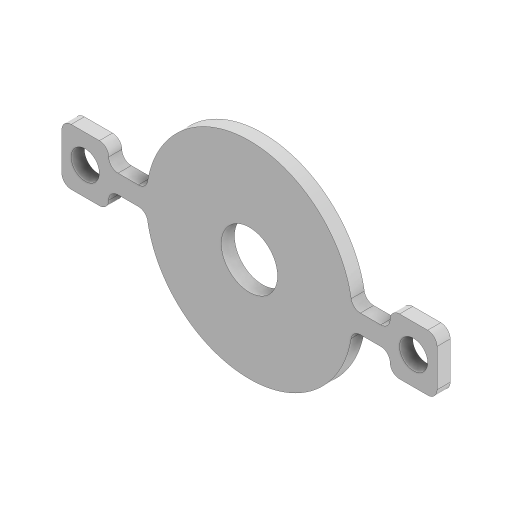
# Autodesk Inventor part: TAPA QUE DESPLAZA CON TORNILLOS
Saved by Autodesk Inventor 2024 (Build 280153000, 153)
## iProperties
Created: 2024-05-26
Part Number: TAPA QUE DESPLAZA CON TORNILLOS
Material: Generic
Document SubType Name: Modeling
Designer: Jhuliams
Density: 1 g/cm^3
Appearance: Default
Author: Jhuliams
Autodesk Inventor part; units mm, degrees
ref_plane "YZ Plane" through (0, 0, 0) normal (1, 0, 0) x (0, 1, 0)
ref_plane "XZ Plane" through (0, 0, 0) normal (0, 1, 0) x (-1, 0, 0)
ref_plane "XY Plane" through (0, 0, 0) normal (0, 0, 1) x (1, 0, 0)
sketch "Sketch1" plane through (0, 0, 0) normal (0, 0, 1) x (1, 0, 0)
  circle A0 centre (0, 0) radius 55
  line L0 (100, 15) -> (100, -15)
  line L1 (10, -15) -> (10, 15)
  line L2 (10, 15) -> (100, -15) construction
  line L3 (100, 15) -> (10, -15) construction
  line L4 (0, 0) -> (0, 20) construction
  line L5 (-100, 15) -> (-100, -15)
  line L6 (-10, -15) -> (-10, 15)
  line L7 (-10, 15) -> (-100, -15) construction
  line L8 (-100, 15) -> (-10, -15) construction
  line L9 (-75, 5) -> (-35, 5)
  line L10 (-35, 5) -> (-35, -5)
  line L11 (-35, -5) -> (-75, -5)
  line L12 (-75, -5) -> (-75, 5)
  line L13 (-75, 5) -> (-35, -5) construction
  line L14 (-35, 5) -> (-75, -5) construction
  line L15 (75, 5) -> (35, 5)
  line L16 (35, 5) -> (35, -5)
  line L17 (35, -5) -> (75, -5)
  line L18 (75, -5) -> (75, 5)
  line L19 (75, 5) -> (35, -5) construction
  line L20 (35, 5) -> (75, -5) construction
  line L21 (-75, 5) -> (-75, 15)
  line L22 (75, 5) -> (75, 15)
  line L23 (-75, -5) -> (-75, -15)
  line L24 (75, -5) -> (75, -15)
  line L25 (10, 15) -> (52.915, 15)
  line L26 (75, 15) -> (100, 15)
  line L27 (100, -15) -> (75, -15)
  line L28 (52.915, -15) -> (10, -15)
  line L29 (-100, -15) -> (-75, -15)
  line L30 (-52.915, -15) -> (-10, -15)
  line L31 (-10, 15) -> (-52.915, 15)
  line L32 (-75, 15) -> (-100, 15)
  point P0 (55, 0)
  point P1 (-55, 0)
  point P2 (54.7723, 5)
  point P3 (54.7723, -5)
  point P4 (-54.7723, -5)
  point P5 (-54.7723, 5)
  dimension "d0" = 110
  dimension "d1" = 90
  dimension "d2" = 30
  dimension "d3" = 20
  dimension "d11" = 40
  dimension "d12" = 10
  constraints: 66 end point, 9 symmetric about line, 7 parallel, 5 point on circle, 5 vertical, 4 midpoint, 3 horizontal, 3 perpendicular, 1 centre point, 1 coincident
  measures "d0" diameter of A0
  measures "d1" distance of L0.end L1.start
  measures "d2" distance of L0.start L0.end
  measures "d3" distance of L4.start L4.end
  measures "d11" distance of L10.end L11.end
  measures "d12" distance of L9.end L10.end
extrude "Extrusion1" add sketch "Sketch1" along normal blind 7
sketch "Sketch2" plane through (0, 0, 7) normal (0, 0, 1) x (1, 0, 0)
  line L0 (0, 0) -> (-87.5, 0) construction
  circle A0 centre (-87.5, 0) radius 7.5
  line L1 (0, 0) -> (0, 20) construction
  circle A1 centre (87.5, 0) radius 7.5
  dimension "d6" = 87.5
  dimension "d7" = 15
  dimension "d8" = 20
  constraints: 4 end point, 2 centre point, 2 coincident, 2 symmetric about line, 1 horizontal, 1 vertical, 1 other
  measures "d6" distance of L0.start L0.end
  measures "d7" diameter of A0
  measures "d8" distance of L0.start L1.end
extrude "Extrusion2" cut sketch "Sketch2" against normal blind 7
fillet "Fillet1" radius 5 16 edges at (-75, -5, 3.5) (-54.7723, -5, 3.5) (-54.7723, 5, 3.5) (-75, 5, 3.5) (-75, -15, 3.5) (-100, -15, 3.5) (-100, 15, 3.5) (-75, 15, 3.5) (54.7723, -5, 3.5) (75, -5, 3.5) (75, -15, 3.5) (100, -15, 3.5) (54.7723, 5, 3.5) (75, 5, 3.5) (75, 15, 3.5) (100, 15, 3.5)
sketch "Sketch4" plane through (0, 0, 7) normal (0, 0, 1) x (1, 0, 0)
  circle A0 centre (0, 0) radius 15
  dimension "d14" = 30
  constraints: 1 centre point, 1 coincident
  measures "d14" diameter of A0
extrude "Extrusion3" cut sketch "Sketch4" against normal blind 10
body "Solid1"
